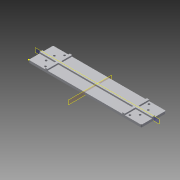
# Autodesk Inventor part: Impact Plate
Saved by Autodesk Inventor 2015 (Build 190159000, 159)
## iProperties
Created: 2016-01-15
Part Number: Impact Plate
Material: ABS Plastic
Document SubType Name: Modeling
Designer: 576994
Mass: 64.2385 g
Surface Area: 282.063 cm^2
Volume: 60.6023 cm^3
Density: 1.06 g/cm^3
Appearance: Smooth - White
Author: 576994
Autodesk Inventor part; units mm, degrees
ref_plane "YZ Plane" through (0, 0, 0) normal (1, 0, 0) x (0, 1, 0)
ref_plane "XZ Plane" through (0, 0, 0) normal (0, 1, 0) x (-1, 0, 0)
ref_plane "XY Plane" through (0, 0, 0) normal (0, 0, 1) x (1, 0, 0)
sketch "Sketch1" plane through (0, 0, 0) normal (0, 0, 1) x (1, 0, 0)
  line L0 (0, 0) -> (235, 0)
  line L1 (235, 0) -> (235, 51)
  line L2 (235, 51) -> (0, 51)
  line L3 (0, 51) -> (0, 0)
  dimension "d0" = 235
  dimension "d1" = 51
  constraints: 8 end point, 2 parallel, 1 horizontal, 1 perpendicular
  measures "d0" distance of L2.end L1.end
  measures "d1" distance of L1.end L0.end
extrude "Extrusion1" add sketch "Sketch1" along normal blind 5
sketch "Sketch2" plane through (0, 0, 5) normal (0, 0, 1) x (1, 0, 0)
  line L0 (0, 0) -> (235, 0)
  line L1 (235, 0) -> (235, 51)
  line L2 (235, 51) -> (0, 51)
  line L3 (0, 51) -> (0, 0)
  line L4 (235, 0) -> (235, 51) projected
  line L5 (0, 22.5) -> (235, 22.5)
  line L6 (235, 22.5) -> (235, 28.5)
  line L7 (235, 28.5) -> (0, 28.5)
  line L8 (0, 28.5) -> (0, 22.5)
  line L9 (0, 22.5) -> (235, 28.5) construction
  line L10 (235, 22.5) -> (0, 28.5) construction
  point P0 (117.5, 25.5)
  dimension "d4" = 6
  constraints: 20 end point, 4 parallel, 2 horizontal, 2 midpoint, 2 perpendicular, 1 point on line
  measures "d4" distance of L6.end L5.end
extrude "Extrusion2" add sketch "Sketch2" along normal blind 3 contours L3 L7 L1 L5
sketch "Sketch3" plane through (0, 0, 5) normal (0, 0, 1) x (1, 0, 0)
  line L0 (0, 28.5) -> (235, 28.5) projected
  line L1 (235, 51) -> (0, 51) projected
  line L2 (34.5, 28.5) -> (39.5, 28.5)
  line L3 (39.5, 28.5) -> (39.5, 51)
  line L4 (39.5, 51) -> (34.5, 51)
  line L5 (34.5, 51) -> (34.5, 28.5)
  point P0 (0, 0)
  dimension "d7" = 5
  constraints: 8 end point, 2 parallel, 2 point on line, 1 horizontal, 1 perpendicular
  measures "d7" distance of L4.end L3.end
sketch "Sketch5" plane through (0, 0, 5) normal (0, 0, 1) x (1, 0, 0)
  line L0 (235, 51) -> (0, 51) projected
  line L1 (117.5, 51) -> (117.5, 0)
  line L2 (235, 28.5) -> (0, 28.5) projected
  line L3 (34.5, 51) -> (39.5, 51)
  line L4 (39.5, 51) -> (39.5, 28.5)
  line L5 (39.5, 28.5) -> (34.5, 28.5)
  line L6 (34.5, 28.5) -> (34.5, 51)
  line L7 (0, 22.5) -> (235, 22.5) projected
  line L8 (34.5, 22.5) -> (39.5, 22.5)
  line L9 (39.5, 22.5) -> (39.5, 0)
  line L10 (39.5, 0) -> (34.5, 0)
  line L11 (34.5, 0) -> (34.5, 22.5)
  line L12 (195.5, 51) -> (195.5, 28.5)
  line L13 (200.5, 28.5) -> (200.5, 51)
  line L14 (195.5, 22.5) -> (195.5, 0)
  line L15 (195.5, 0) -> (200.5, 0)
  line L16 (200.5, 0) -> (200.5, 22.5)
  line L17 (195.5, 28.5) -> (200.5, 28.5)
  line L18 (195.5, 22.5) -> (200.5, 22.5)
  line L19 (195.5, 51) -> (200.5, 51)
  point P0 (0, 0)
  dimension "d13" = 5
  constraints: 34 end point, 8 symmetric about line, 4 parallel, 3 perpendicular, 3 point on line, 2 collinear, 2 horizontal, 1 midpoint, 1 vertical
  measures "d13" distance of L4.end L5.end
extrude "Extrusion5" add sketch "Sketch3" along normal blind 3
extrude "Extrusion6" add sketch "Sketch5" along normal blind 3 contours L9 L10 L11 L7
extrude "Extrusion7" add sketch "Sketch5" along normal blind 3 contours L13 L2 L12 L0 | L7 L16 L15 L14
sketch "Sketch8" plane through (0, 0, 5) normal (0, 0, 1) x (1, 0, 0)
  circle A0 centre (29.5, 5.625) radius 1.6
  circle A1 centre (19.5, 16.875) radius 1.6
  line L0 (39.5, 0) -> (39.5, 22.5) projected
  line L1 (34.5, 22.5) -> (34.5, 0) projected
  line L2 (0, 0) -> (34.5, 0) projected
  dimension "d24" = 3.2
  dimension "d25" = 3.2
  dimension "d27" = 5
  dimension "d28" = 5.625
  dimension "d29" = 15
  dimension "d30" = 16.875
  constraints: 2 centre point
  measures "d24" diameter of A0
  measures "d25" diameter of A1
  measures "d27" distance from line of A0.centre L1
  measures "d28" distance from line of A0.centre L2
  measures "d29" distance from line of L1 A1.centre
  measures "d30" distance from line of L2 A1.centre
extrude "Extrusion9" cut sketch "Sketch8" against normal blind 10
sketch "Sketch9" plane through (0, 0, 8) normal (0, 0, 1) x (1, 0, 0)
  line L0 (0, 51) -> (0, 0) projected
  line L1 (0, 25.5) -> (235, 25.5)
  line L2 (235, 0) -> (235, 51) projected
  line L3 (117.5, 25.5) -> (117.5, -30.3106)
  constraints: 4 end point, 3 midpoint, 1 vertical
ref_plane "Work Plane1" through (0, 25.5, 8) normal (0, 1, 0) x (1, 0, 0)
mirror "Mirror1" about plane through (0, 25.5, 8) normal (0, 1, 0) of "Extrusion9"
ref_plane "Work Plane2" through (117.5, 25.5, 8) normal (1, 0, 0) x (0, -1, 0)
mirror "Mirror2" about plane through (117.5, 25.5, 8) normal (1, 0, 0) of "Extrusion9", "Mirror1"
sketch "Sketch11" plane through (0, 0, 5) normal (0, 0, 1) x (1, 0, 0)
  circle A0 centre (19.5, 16.875) radius 1.6 projected
  circle A1 centre (19.5, 16.875) radius 2.1
  circle A2 centre (29.5, 5.625) radius 1.6 projected
  circle A3 centre (29.5, 5.625) radius 2.1
  point P0 (0, 0)
  dimension "d35" = 4.2
  dimension "d36" = 4.2
  constraints: 2 centre point, 2 coincident
  measures "d35" diameter of A1
  measures "d36" diameter of A3
extrude "Extrusion10" cut sketch "Sketch11" against normal blind 10 contours A0 | A1 | A2 | A3
mirror "Mirror3" about plane through (0, 25.5, 8) normal (0, 1, 0) of "Extrusion10"
mirror "Mirror4" about plane through (117.5, 25.5, 8) normal (1, 0, 0) of "Extrusion10", "Mirror3"
fillet "Fillet1" radius 2 4 edges at (235, 51, 2.5) (0, 51, 2.5) (0, 0, 2.5) (235, 0, 2.5)
sketch "Sketch12" plane through (0, 0, 5) normal (0, 0, 1) x (1, 0, 0)
  point P0 (0, 0)
body "Solid1"
